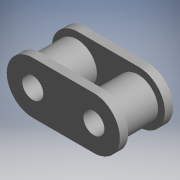
# Autodesk Inventor part: 06B - 1 RP - Body
Saved by Autodesk Inventor 2019 (Build 230136000, 136)
## iProperties
Category: PARTsolutions
Company: KANA
Part Number: 06B - 1 RP - Body
Material: 一般
Catalog Web Link: www.cadenas.de
Description: Standard Chain_Body1-
Vendor: KANA
Document SubType Name: Modeling
Designer: partserver
Manufacturer: KANA
Mass: 0.554581 g
Surface Area: 9.06714 cm^2
Volume: 0.554581 cm^3
Density: 1 g/cm^3
Appearance: PSOLRGB-192-192-192
PSOL_IDENT_0: {$CADENAS_DATA\23d-libs\kana\roller_chain\standard_chain\standard_chain_body1.prj},188 {VTYP=3D},{NB=
PSOL_IDENT_1: 06B - 1 RP - Body},{LINA=06B - 1 RP},{NN=Standard Chain_Body1},{DATE=04.07.2018 01:10:23},{GEOMDATE=
PSOL_IDENT_2: 05.10.2016 10:19:00},{VERSION=},{LINEID=250},{WBVAR=NOL},{WBNUMERIC=NOL}  {NB=06B - 1 RP - Body},{LI
PSOL_IDENT_3: NA=06B - 1 RP},{KT=DUMMY},{CNO=06B},{PT=RP},{NOL=1},{NOLX=1},{P=9.525},{R=6.350},{W=5.720},{T=1.300}
PSOL_IDENT_4: ,{H=8.100},{D=3.280},{L=13.6},{C=10.24}
NB: 06B - 1 RP - Body
NN: Standard Chain_Body1
NBSYN: $CNO. - $NOL. $PT. - Body
LINA: 06B - 1 RP
CATALOG: KANA
CNO: 06B
PT: RP
NOL: 1
P: 9.525
R: 6.35
W: 5.72
T: 1.3
H: 8.1
D: 3.28
SUPPLIER: KANA
ARTICLENO: 06B - 1 RP - Body
BOMINFO: 06B - 1 RP
CREATOR: CADENAS GmbH
Title: 06B - 1 RP
Author: Cadenas PARTsolutions
Autodesk Inventor part; units mm, degrees
sketch "Sketch_2" plane through (0, 0, 0) normal (0, 0, 1) x (1, 0, 0)
  line L0 (0, -2.86) -> (0, 2.86)
  line L1 (1.64, 2.86) -> (1.64, -2.86)
  line L2 (1.64, -2.86) -> (2.8575, -2.86)
  arc A0 (2.8575, -2.86) -> (3.175, -2.5425) centre (2.8575, -2.5425) ccw
  line L3 (3.175, -2.5425) -> (3.175, 2.5425)
  arc A1 (3.175, 2.5425) -> (2.8575, 2.86) centre (2.8575, 2.5425) ccw
  line L4 (2.8575, 2.86) -> (1.64, 2.86)
  constraints: 10 end point, 4 point on circle, 2 centre point
revolve "Revolution1" add sketch "Sketch_2" angle 360 about axis through (0, -2.86, 0) along (0, -1, 0)
sketch "Sketch_5" plane through (0, 2.86, 0) normal (0, 1, 0) x (1, 0, 0)
  arc A0 (0, 4.05) -> (0, -4.05) centre (0, 0) ccw
  line L0 (0, -4.05) -> (9.525, -4.05)
  arc A1 (9.525, -4.05) -> (9.525, 4.05) centre (9.525, 0) ccw
  line L1 (9.525, 4.05) -> (0, 4.05)
  circle A2 centre (9.525, 0) radius 1.64
  circle A3 centre (0, 0) radius 1.64
  constraints: 4 centre point, 4 end point, 4 point on circle
extrude "Extrusion1" add sketch "Sketch_5" along normal blind 1.3
sketch "Sketch_6" plane through (0, -2.86, 0) normal (0, 1, 0) x (1, 0, 0)
  arc A0 (0, 4.05) -> (0, -4.05) centre (0, 0) ccw
  line L0 (0, -4.05) -> (9.525, -4.05)
  arc A1 (9.525, -4.05) -> (9.525, 4.05) centre (9.525, 0) ccw
  line L1 (9.525, 4.05) -> (0, 4.05)
  circle A2 centre (9.525, 0) radius 1.64
  circle A3 centre (0, 0) radius 1.64
  constraints: 4 centre point, 4 end point, 4 point on circle
extrude "Extrusion2" add sketch "Sketch_6" against normal blind 1.3
sketch "Sketch_8" plane through (0, 0, 0) normal (0, 0, 1) x (1, 0, 0)
  line L0 (9.525, -2.86) -> (9.525, 2.86)
  line L1 (11.165, 2.86) -> (11.165, -2.86)
  line L2 (11.165, -2.86) -> (12.3825, -2.86)
  arc A0 (12.3825, -2.86) -> (12.7, -2.5425) centre (12.3825, -2.5425) ccw
  line L3 (12.7, -2.5425) -> (12.7, 2.5425)
  arc A1 (12.7, 2.5425) -> (12.3825, 2.86) centre (12.3825, 2.5425) ccw
  line L4 (12.3825, 2.86) -> (11.165, 2.86)
  constraints: 10 end point, 4 point on circle, 2 centre point
revolve "Revolution2" add sketch "Sketch_8" angle 360 about axis through (9.525, -2.86, 0) along (0, -1, 0)
ref_plane "for_body1_a_XY" through (9.525, 0, 0) normal (0, 1, 0) x (1, 0, 0)
ref_plane "for_body1_a_YZ" through (9.525, 0, 0) normal (1, 0, 0) x (0, 0, -1)
ref_plane "for_body1_a_ZX" through (9.525, 0, 0) normal (0, 0, -1) x (0, 1, 0)
ref_plane "to_dummy_XY" through (0, 0, 0) normal (0, 1, 0) x (1, 0, 0)
ref_plane "to_dummy_YZ" through (0, 0, 0) normal (1, 0, 0) x (0, 0, -1)
ref_plane "to_dummy_ZX" through (0, 0, 0) normal (0, 0, -1) x (0, 1, 0)
body "Solid1"
